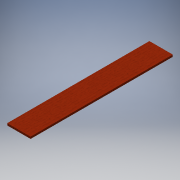
# Autodesk Inventor part: Wine Glass Holder Middle
Saved by Autodesk Inventor 2016 (Build 200138000, 138)
## iProperties
Created: 2017-10-31
Part Number: Wine Glass Holder Middle
Material: Generic
Document SubType Name: Modeling
Designer: mathaetaes
Density: 1 g/cm^3
Appearance: Default
Author: mathaetaes
Autodesk Inventor part; units mm, degrees
ref_plane "YZ Plane" through (0, 0, 0) normal (1, 0, 0) x (0, 1, 0)
ref_plane "XZ Plane" through (0, 0, 0) normal (0, 1, 0) x (-1, 0, 0)
ref_plane "XY Plane" through (0, 0, 0) normal (0, 0, 1) x (1, 0, 0)
sketch "Sketch1" plane through (0, 0, 0) normal (0, 0, 1) x (1, 0, 0)
  line L0 (-71.9423, -10.5563) -> (4.2577, -10.5563)
  line L1 (4.2577, -10.5563) -> (4.2577, -16.9063)
  line L2 (4.2577, -16.9063) -> (-71.9423, -16.9063)
  line L3 (-71.9423, -16.9063) -> (-71.9423, -10.5563)
  point P0 (0, 0)
  dimension "d0" = 76.2
  dimension "d1" = 6.35
  constraints: 8 end point, 2 parallel, 1 horizontal, 1 perpendicular
  measures "d0" distance of L1.end L2.end
  measures "d1" distance of L0.end L1.end
extrude "Extrusion1" add sketch "Sketch1" along normal blind 463.55
body "Solid1"
